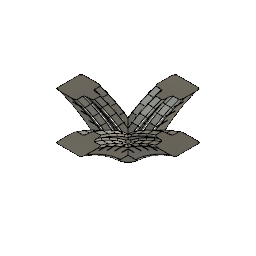
bear_overhang_50-70 (Autodesk Fusion 360 design; units mm, degrees)
Autodesk Fusion 360 part; units mm, degrees
note: some values were not read from the file. Chosen so that the rebuilt part matches the saved one: which sketch regions a step uses; which pieces of a blend or face edit are solid.
sketch "arm" plane through (0, 0, 0) normal (0, 1, 0) x (1, 0, 0) in component "bear_overhang"
  line L0 (15.4713, 0) -> (0, 0)
  line L1 (24.8557, -7.2) -> (30.0519, -10.2)
  line L2 (15.4713, 0) -> (20, -3.8)
  line L3 (20, -3.8) -> (24.8557, -7.2)
  line L4 (0, -3.8) -> (0, 0)
  line L5 (0, 0) -> (0, -27.1786) construction
  line L6 (41.1225, -14.8) -> (27.1225, -14.8)
  line L7 (16.0519, -10.2) -> (10.8557, -7.2)
  line L8 (30.0519, -10.2) -> (16.0519, -10.2) construction
  line L9 (24.8557, -7.2) -> (10.8557, -7.2) construction
  line L10 (20, -3.8) -> (6, -3.8) construction
  line L11 (10.8557, -7.2) -> (6, -3.8)
  line L12 (6, -3.8) -> (1.4713, 0)
  line L13 (27.1225, -14.8) -> (21.1225, -14.8)
  line L14 (10.0519, -10.2) -> (4.8557, -7.2)
  line L15 (4.8557, -7.2) -> (0, -3.8)
  line L16 (30.0519, -10.2) -> (35.6276, -12.8)
  line L17 (35.6276, -12.8) -> (41.1225, -14.8)
  line L18 (16.0519, -10.2) -> (21.6276, -12.8)
  line L19 (21.6276, -12.8) -> (27.1225, -14.8)
  line L20 (10.0519, -10.2) -> (15.6276, -12.8)
  line L21 (15.6276, -12.8) -> (21.1225, -14.8)
  line L22 (35.6276, -12.8) -> (21.6276, -12.8) construction
  line L23 (0, -3.8) -> (6, -3.8)
  dimension "d9" = 3.8
  dimension "d10" = 3.4
  dimension "d13" = 3
  dimension "d17" = 14
  dimension "d24" = 50
  dimension "d25" = 55
  dimension "d26" = 60
  dimension "d33" = 6
  dimension "d45" = 7.6
  dimension "d46" = 7.6019
  dimension "d50" = 65
  dimension "d51" = 70
  dimension "d52" = 2.6
  dimension "d53" = 2
  dimension "d54" = 6.6254
  dimension "d55" = 7.0171
  dimension "d78" = 14
  constraint horizontal L6
  constraint horizontal L8
  constraint equal L6 L8
  constraint horizontal L9
  constraint equal L6 L9
  constraint equal L6 L10
  constraint horizontal L10
  constraint parallel L6 L13
  constraint coincident L8 L14.start
  constraint horizontal L0
  constraint coincident L9 L14.end
  constraint coincident L10 L4.start
  constraint parallel L11 L15
  constraint parallel L7 L14
  constraint coincident L0.end L4.end
  constraint horizontal L22
  constraint equal L6 L22
  constraint parallel L18 L20
  constraint coincident L20.end L22
  constraint parallel L19 L21
  constraint perpendicular L0 L5
  constraint perpendicular L0 L4
  constraint coincident L0 L12.end
  measures "d9" vertical distance of L2.end L0.start
  measures "d10" vertical distance of L2.end L1.start
  measures "d13" vertical distance of L1.end L1.start
  measures "d17" distance of L6.start L6.end
  measures "d24" angle of L2 L5
  measures "d25" angle of L3 L5
  measures "d26" angle of L1 L5
  measures "d33" distance of L6.end L13.end
  measures "d50" angle of L5 L16
  measures "d51" angle of L5 L17
  measures "d52" vertical distance of L1.end L16.end
  measures "d53" vertical distance of L6.start L16.end
  measures "d78" distance of L0.start L12.end
extrude "Extrude1" add sketch "arm" along normal mid plane 18 contours L0 L1 L2 L3 L6 L7 L11 L12 L16 L17 L18 L19 | L0 L4 L12 L23 makes body 1 in component "bear_overhang"
extrude "Extrude2" add sketch "arm" along normal mid plane 6 contours L0 L1 L2 L3 L6 L7 L11 L12 L16 L17 L18 L19 | L7 L11 L13 L14 L15 L18 L19 L20 L21 L23 bodies 1 in component "bear_overhang"
fillet "Fillet1" radius 1 34 edges at (8.4279, -9, 5.5) (13.4538, -9, 8.7) (17.7357, -9, 1.9) (22.4279, -9, 5.5) (27.4538, -9, 8.7) (8.4279, -3, 5.5) (13.4538, -3, 8.7) (27.4538, 9, 8.7) (22.4279, 9, 5.5) (17.7357, 9, 1.9) (8.4279, 9, 5.5) (13.4538, 9, 8.7) (13.4538, 3, 8.7) (8.4279, 3, 5.5) (2.4279, 3, 5.5) (7.4538, 3, 8.7) (2.4279, -3, 5.5) (7.4538, -3, 8.7) (32.8397, -9, 11.5) (38.3751, -9, 13.8) (24.3751, -9, 13.8) (18.8397, -9, 11.5) (18.8397, -3, 11.5) (24.3751, -3, 13.8) (18.3751, -3, 13.8) (12.8397, -3, 11.5) (12.8397, 3, 11.5) (18.3751, 3, 13.8) (18.8397, 9, 11.5) (24.3751, 9, 13.8) (38.3751, 9, 13.8) (32.8397, 9, 11.5) (24.3751, 3, 13.8) (18.8397, 3, 11.5) on bodies 1 in component "bear_overhang"
sketch "angle_indication" plane through (0, -9, 0) normal (0, -1, 0) x (1, 0, 0) in component "bear_overhang"
  line L0 (20, 3.8) -> (6, 3.8)
  line L1 (24.8557, 7.2) -> (10.8557, 7.2)
  line L2 (30.0519, 10.2) -> (16.0519, 10.2)
  line L3 (35.6276, 12.8) -> (21.6276, 12.8)
  line L4 (13, 3.8) -> (13.2856, 4)
  line L5 (13.2856, 4) -> (6.2856, 4)
  line L6 (17.8557, 7.2) -> (18.2021, 7.4)
  line L7 (18.2021, 7.4) -> (11.2021, 7.4)
  line L8 (23.0519, 10.2) -> (23.4808, 10.4)
  line L9 (23.4808, 10.4) -> (16.4808, 10.4)
  line L10 (28.6276, 12.8) -> (29.1771, 13)
  line L11 (29.1771, 13) -> (22.1771, 13)
  line L12 (10.8557, 7.2) -> (6, 3.8)
  line L13 (16.0519, 10.2) -> (10.8557, 7.2)
  line L14 (21.6276, 12.8) -> (16.0519, 10.2)
  line L15 (27.1225, 14.8) -> (21.6276, 12.8)
  point P0 (20, 3.8)
  point P1 (24.8557, 7.2)
  point P2 (30.0519, 10.2)
  point P3 (35.6276, 12.8)
  point P4 (15.4713, 0)
  dimension "d68" = 0.2
  dimension "d69" = 0.2
  dimension "d70" = 0.2
  dimension "d71" = 0.2
  constraint midpoint L0 L4.start
  constraint midpoint L1 L6.start
  constraint midpoint L2 L8.start
  constraint midpoint L3 L10.start
  constraint parallel L0 L5
  constraint parallel L1 L7
  constraint parallel L2 L9
  constraint parallel L3 L11
  constraint coincident L11.end L15
  constraint coincident L3.end L14.start
  constraint coincident L2.end L13.start
  constraint coincident L1.end L12.start
  constraint coincident L0.end L12.end
  constraint coincident P0 L0.start
  constraint coincident P1 L1.start
  constraint coincident P2 L2.start
  constraint coincident P3 L3.start
  constraint parallel L4 L12
  constraint parallel L6 L13
  constraint parallel L8 L14
  constraint parallel L10 L15
  constraint coincident L9.end L14
  constraint coincident L7.end L13
  constraint coincident L5.end L12
  measures "d68" distance of L0 L5
  measures "d69" distance of L1 L7
  measures "d70" distance of L2 L9
  measures "d71" distance of L3 L11
extrude "Extrude2'" cut sketch "angle_indication" against normal blind 0.3 bodies 1 in component "bear_overhang"
mirror "Mirror1" about plane through (0, 0, 0) normal (0, 1, 0) of "Extrude2'" in component "bear_overhang"
pattern_circular "C-Pattern1" count 4 over 360 about axis through (0, 0, 1.75) along (0, 0, 1) of bodies 1 makes body 2 at (-1.2793, 34.4938, 14.8) makes body 3 at (-34.4938, -1.2793, 14.8) makes body 4 at (1.2793, -34.4938, 14.8) in component "bear_overhang"
combine "Combine1" operation add target body 1 tool bodies 2 3 4 in component "bear_overhang"
sketch "orientation_mark" plane through (0, 0, 0) normal (0, 0, -1) x (1, 0, 0) in component "bear_overhang"
  line L0 (-9, 9) -> (-13.9156, 9)
  line L1 (-13.9156, -9) -> (-9, -9)
  line L2 (-9, -9) -> (-9, -13.9156)
  line L3 (9, -13.9156) -> (9, -9)
  line L4 (9, -9) -> (13.9156, -9)
  line L5 (13.9156, 9) -> (9, 9)
  line L6 (9, 9) -> (9, 13.9156)
  line L7 (-9, 13.9156) -> (-9, 9)
  line L8 (-9, 9) -> (9, 9) construction
  line L9 (0, 9) -> (0, 15.4713) construction
  circle A0 centre (0, 12.2357) radius 1.5
  arc A1 (8, -15.4713) -> (15.4713, -8) centre (8, -8) ccw
  arc A2 (15.4713, 8) -> (8, 15.4713) centre (8, 8) ccw
  arc A3 (-8, 15.4713) -> (-15.4713, 8) centre (-8, 8) ccw
  arc A4 (-15.4713, -8) -> (-8, -15.4713) centre (-8, -8) ccw
  ellipse E0 centre (-13.9156, 8) end of major axis (-15.4713, 8) minor radius 1 (-13.9156, 9) -> (-15.4713, 8) ccw construction
  line L10 (-15.4713, 8) -> (-15.4713, -8)
  ellipse E1 centre (-13.9156, -8) end of major axis (-15.4713, -8) minor radius 1 (-15.4713, -8) -> (-13.9156, -9) ccw construction
  ellipse E2 centre (-8, -13.9156) end of major axis (-8, -15.4713) minor radius 1 (-9, -13.9156) -> (-8, -15.4713) ccw construction
  line L11 (-8, -15.4713) -> (8, -15.4713)
  ellipse E3 centre (8, -13.9156) end of major axis (8, -15.4713) minor radius 1 (8, -15.4713) -> (9, -13.9156) ccw construction
  ellipse E4 centre (13.9156, -8) end of major axis (15.4713, -8) minor radius 1 (13.9156, -9) -> (15.4713, -8) ccw construction
  line L12 (15.4713, -8) -> (15.4713, 8)
  ellipse E5 centre (13.9156, 8) end of major axis (15.4713, 8) minor radius 1 (15.4713, 8) -> (13.9156, 9) ccw construction
  ellipse E6 centre (8, 13.9156) end of major axis (8, 15.4713) minor radius 1 (9, 13.9156) -> (8, 15.4713) ccw construction
  line L13 (8, 15.4713) -> (-8, 15.4713)
  ellipse E7 centre (-8, 13.9156) end of major axis (-8, 15.4713) minor radius 1 (-8, 15.4713) -> (-9, 13.9156) ccw construction
  dimension "d56" = 3
  constraint coincident L0.start L7.end
  constraint coincident L5.end L6.start
  constraint midpoint L8 L9.start
  constraint midpoint L9 A0.centre
  constraint coincident A4.end L11.start
  constraint coincident A4.start L10.end
  constraint coincident A3.end L10.start
  constraint coincident A3.start L13.end
  constraint coincident A2.end L13.start
  constraint coincident A1.end L12.start
  constraint coincident A1.start L11.end
  constraint tangent A1 L11
  constraint tangent A4 L11
  constraint tangent A3 L10
  constraint tangent A2 L13
  constraint midpoint L9.end L13
  constraint coincident A2.start L12.end
  measures "d56" diameter of A0
extrude "Extrude1'" cut sketch "orientation_mark" against normal blind 0.6 contours A0 bodies 1 in component "bear_overhang"
extrude "Extrude3" add sketch "orientation_mark" against normal blind 0.2 bodies 1 in component "bear_overhang"
component "bear_overhang" placed x (1, 0, 0) y (0, 1, 0) z (0, 0, 1) at (0, 0, 0)
equation "d9 = layer_height * 19"
equation "d10 = layer_height * 17"
equation "d13 = layer_height * 15"
equation "d17 = arm_layer_length"
equation "d31 = arm_width"
equation "d33 = 20 mm - arm_layer_length"
equation "d34 = arm_support_width"
equation "layer_height = 0.2 mm"
equation "arm_width = 18 mm"
equation "arm_support_width = arm_width / 3"
equation "d52 = layer_height * 13"
equation "d53 = layer_height * 10"
equation "d57 = -layer_height * 3"
equation "arm_layer_length = 14 mm"
equation "d68 = layer_height"
equation "d69 = layer_height"
equation "d70 = layer_height"
equation "d71 = layer_height"
equation "d75 = -layer_height"
equation "d78 = arm_layer_length"
named bodies: "Body1 (1)"
